Autodesk Fusion 360 part; units mm, degrees
(part 2 of 2)
  line L93 (-101.7927, 9.6669) -> (-102.2055, 10.4133)
  spline S43 degree 3 poles (-102.1987, 11.9336) (-102.3688, 11.6535) (-102.4812, 11.4913) (-102.5578, 11.3159) (-102.5705, 11.2723) (-102.5795, 11.182) (-102.5739, 11.1357) (-102.5157, 10.943) (-102.3981, 10.7613) (-102.2055, 10.4133) knots -0.305228 -0.305228 -0.305228 -0.305228 -0.202643 -0.202643 -0.163031 -0.163031 -0.119338 -0.119338 0 0 0 0
  line L94 (-102.1987, 11.9336) -> (-101.779, 12.625)
  line L95 (-101.779, 12.625) -> (-100.2331, 12.625)
  line L96 (-100.2331, 12.625) -> (-100.2331, 6.4783)
  spline S44 degree 3 poles (-78.8802, 8.0397) (-78.8802, 8.0397) (-78.8802, 8.0397) (-78.8801, 8.0397) (-78.8801, 8.0397) (-78.88, 8.0397) (-78.88, 8.0398) (-78.8798, 8.04) (-78.8797, 8.0402) (-78.8794, 8.041) (-78.8792, 8.0418) (-78.8786, 8.045) (-78.8782, 8.0484) (-78.8769, 8.0615) (-78.8761, 8.0763) (-78.8737, 8.1251) (-78.8722, 8.1818) (-78.8679, 8.3654) (-78.8655, 8.5656) (-78.8591, 9.2073) (-78.8573, 9.8073) (-78.8573, 10.3314) knots -0.220445 -0.220445 -0.220445 -0.220445 -0.220429 -0.220429 -0.220411 -0.220411 -0.220367 -0.220367 -0.220257 -0.220257 -0.219969 -0.219969 -0.219065 -0.219065 -0.216007 -0.216007 -0.203797 -0.203797 -0.157247 -0.157247 0 0 0 0
  spline S45 degree 3 poles (-79.66, 9.1105) (-79.3146, 8.6225) (-79.0132, 8.2063) (-78.9036, 8.0659) (-78.8903, 8.0491) (-78.8828, 8.0415) (-78.8818, 8.0406) (-78.8809, 8.0399) (-78.8807, 8.0398) (-78.8804, 8.0397) (-78.8803, 8.0397) (-78.8802, 8.0397) knots -0.01704 -0.01704 -0.01704 -0.01704 -0.001899 -0.001899 -0.000322 -0.000322 -0.000087 -0.000087 -0.000024 -0.000024 0 0 0 0
  line L97 (-79.66, 9.1105) -> (-80.4169, 10.1795)
  line L98 (-80.4169, 10.1795) -> (-80.4169, 12.6249)
  line L99 (-80.4169, 12.6249) -> (-78.8573, 12.6249)
  line L100 (-78.8573, 12.6249) -> (-78.8573, 10.3314)
  line L101 (-114.2466, 6.4942) -> (-115.0035, 6.4594)
  line L102 (-115.0035, 6.4594) -> (-115.0035, 7.2486)
  line L103 (-115.0035, 7.2486) -> (-115.0035, 8.0379)
  line L104 (-115.0035, 8.0379) -> (-114.5448, 8.0379)
  spline S46 degree 3 poles (-114.0861, 8.2672) (-114.0861, 8.2225) (-114.0874, 8.1854) (-114.0972, 8.1399) (-114.102, 8.1261) (-114.1159, 8.1022) (-114.1245, 8.0925) (-114.1483, 8.0745) (-114.1646, 8.0667) (-114.2516, 8.0407) (-114.362, 8.0379) (-114.5448, 8.0379) knots -0.128591 -0.128591 -0.128591 -0.128591 -0.100749 -0.100749 -0.086063 -0.086063 -0.071871 -0.071871 -0.054849 -0.054849 0 0 0 0
  spline S47 degree 3 poles (-113.2956, 8.4966) (-113.6377, 8.4966) (-113.8328, 8.4962) (-113.9744, 8.4707) (-113.9988, 8.4635) (-114.0318, 8.4477) (-114.0428, 8.44) (-114.0608, 8.4218) (-114.0676, 8.411) (-114.0856, 8.3666) (-114.0861, 8.3239) (-114.0861, 8.2672) knots -0.067797 -0.067797 -0.067797 -0.067797 -0.038062 -0.038062 -0.029608 -0.029608 -0.023495 -0.023495 -0.017016 -0.017016 0 0 0 0
  line L105 (-113.2956, 8.4966) -> (-112.5051, 8.4966)
  line L106 (-112.5051, 8.4966) -> (-112.543, 7.9012)
  spline S48 degree 3 poles (-114.2466, 6.4942) (-114.0442, 6.5035) (-113.8242, 6.522) (-113.4498, 6.5931) (-113.2959, 6.6391) (-113.052, 6.759) (-112.9528, 6.8282) (-112.7761, 7.0176) (-112.7103, 7.133) (-112.5965, 7.4348) (-112.5592, 7.6462) (-112.543, 7.9012) knots -0.314262 -0.314262 -0.314262 -0.314262 -0.243332 -0.243332 -0.182489 -0.182489 -0.132108 -0.132108 -0.076683 -0.076683 0 0 0 0
  line L107 (-103.9945, 6.4783) -> (-105.5541, 6.4783)
  line L108 (-105.5541, 6.4783) -> (-105.5511, 11.8451)
  line L109 (-105.5511, 11.8451) -> (-103.9945, 8.869)
  line L110 (-103.9945, 8.869) -> (-103.9945, 6.4783)
  line L111 (-79.6205, 6.4783) -> (-80.3728, 6.4783)
  line L112 (-80.3728, 6.4783) -> (-82.2755, 9.1431)
  spline S49 degree 3 poles (-84.1783, 12.22) (-84.1783, 12.1228) (-84.1718, 12.0391) (-84.0959, 11.8191) (-84.0269, 11.6832) (-83.6449, 11.0655) (-83.1484, 10.3655) (-82.2755, 9.1431) knots -0.89304 -0.89304 -0.89304 -0.89304 -0.671781 -0.671781 -0.450601 -0.450601 0 0 0 0
  line L113 (-84.1783, 12.22) -> (-84.1783, 12.6321)
  line L114 (-84.1783, 12.6321) -> (-83.3779, 12.6056)
  line L115 (-83.3779, 12.6056) -> (-82.5774, 12.5791)
  line L116 (-82.5774, 12.5791) -> (-80.7274, 9.9771)
  spline S50 degree 3 poles (-79.6205, 6.4783) (-79.3917, 6.4783) (-79.203, 6.4838) (-79.0027, 6.5232) (-78.949, 6.5392) (-78.8759, 6.5766) (-78.8498, 6.5945) (-78.8078, 6.6384) (-78.7925, 6.6625) (-78.7689, 6.7242) (-78.7644, 6.7611) (-78.7658, 6.8517) (-78.7776, 6.9137) (-78.9459, 7.4456) (-79.5495, 8.3203) (-80.7274, 9.9771) knots -1.178058 -1.178058 -1.178058 -1.178058 -0.964403 -0.964403 -0.875567 -0.875567 -0.82025 -0.82025 -0.769095 -0.769095 -0.704441 -0.704441 -0.609856 -0.609856 0 0 0 0
  line L117 (-62.7108, 11.0653) -> (-64.2704, 11.0653)
  line L118 (-64.2704, 11.0653) -> (-64.2704, 12.6249)
  line L119 (-64.2704, 12.6249) -> (-62.7108, 12.6249)
  line L120 (-62.7108, 12.6249) -> (-62.7108, 11.0653)
  line L121 (-85.4023, 6.4783) -> (-86.1675, 6.4783)
  line L122 (-86.1675, 6.4783) -> (-87.0995, 9.4403)
  spline S51 degree 3 poles (-87.2699, 12.625) (-87.4394, 12.625) (-87.5787, 12.6376) (-87.7375, 12.6363) (-87.7813, 12.6329) (-87.839, 12.6184) (-87.8597, 12.6108) (-87.894, 12.5891) (-87.9073, 12.5767) (-87.9308, 12.5439) (-87.9401, 12.5226) (-87.9545, 12.4632) (-87.9573, 12.4213) (-87.9358, 12.0193) (-87.6604, 11.2232) (-87.0995, 9.4403) knots -1.159539 -1.159539 -1.159539 -1.159539 -0.929801 -0.929801 -0.821044 -0.821044 -0.758836 -0.758836 -0.705055 -0.705055 -0.643157 -0.643157 -0.560713 -0.560713 0 0 0 0
  line L123 (-87.2699, 12.625) -> (-86.5083, 12.625)
  line L124 (-86.5083, 12.625) -> (-85.5727, 9.6479)
  spline S52 degree 3 poles (-84.637, 6.5745) (-84.637, 6.6129) (-84.8584, 7.3414) (-85.1118, 8.1738) (-85.3556, 8.9573) (-85.5727, 9.6479) knots -0.275208 -0.275208 -0.275208 -0.275208 -0.21716 -0.21716 0 0 0 0
  spline S53 degree 3 poles (-85.4023, 6.4783) (-85.1852, 6.4783) (-85.0047, 6.4859) (-84.8145, 6.507) (-84.7429, 6.5172) (-84.6801, 6.5376) (-84.666, 6.5432) (-84.6509, 6.5528) (-84.6464, 6.5562) (-84.6411, 6.5623) (-84.6395, 6.5648) (-84.6375, 6.5698) (-84.637, 6.5721) (-84.637, 6.5745) knots -0.053648 -0.053648 -0.053648 -0.053648 -0.020754 -0.020754 -0.006983 -0.006983 -0.003161 -0.003161 -0.001603 -0.001603 -0.000721 -0.000721 0 0 0 0
  line L125 (-45.0964, 6.4783) -> (-48.5826, 6.4783)
  line L126 (-48.5826, 6.4783) -> (-48.5826, 8.0379)
  line L127 (-48.5826, 8.0379) -> (-45.0964, 8.0379)
  line L128 (-45.0964, 8.0379) -> (-45.0964, 6.4783)
  line L129 (-115.3705, 6.4783) -> (-115.9897, 6.4865)
  spline S54 degree 3 poles (-116.9301, 6.5861) (-116.8418, 6.561) (-116.6918, 6.5372) (-116.3514, 6.5012) (-116.1605, 6.4888) (-115.9897, 6.4865) knots -0.102601 -0.102601 -0.102601 -0.102601 -0.051231 -0.051231 0 0 0 0
  spline S55 degree 3 poles (-117.8471, 9.57) (-117.8473, 8.4438) (-117.8321, 7.7752) (-117.7062, 7.2163) (-117.6651, 7.1041) (-117.5648, 6.9297) (-117.5053, 6.8604) (-117.3031, 6.7061) (-117.1405, 6.6459) (-116.9301, 6.5861) knots -0.278348 -0.278348 -0.278348 -0.278348 -0.149693 -0.149693 -0.105736 -0.105736 -0.065646 -0.065646 0 0 0 0
  spline S56 degree 3 poles (-116.1845, 12.6085) (-116.5349, 12.5917) (-116.8146, 12.5695) (-117.1517, 12.4821) (-117.2527, 12.4421) (-117.4251, 12.3326) (-117.4945, 12.2657) (-117.621, 12.084) (-117.6743, 11.9601) (-117.8311, 11.3627) (-117.847, 10.6695) (-117.8471, 9.57) knots -0.833641 -0.833641 -0.833641 -0.833641 -0.642856 -0.642856 -0.543072 -0.543072 -0.446446 -0.446446 -0.329868 -0.329868 0 0 0 0
  line L130 (-116.1845, 12.6085) -> (-115.3705, 12.6474)
  line L131 (-115.3705, 12.6474) -> (-115.3705, 11.0653)
  line L132 (-115.3705, 11.0653) -> (-116.2879, 11.0653)
  line L133 (-116.2879, 11.0653) -> (-116.2879, 8.0379)
  line L134 (-116.2879, 8.0379) -> (-115.3705, 8.0379)
  line L135 (-115.3705, 8.0379) -> (-115.3705, 6.4783)
  line L136 (-45.0964, 11.0653) -> (-48.5826, 11.0653)
  line L137 (-48.5826, 11.0653) -> (-48.5826, 12.6249)
  line L138 (-48.5826, 12.6249) -> (-45.0964, 12.6249)
  line L139 (-45.0964, 12.6249) -> (-45.0964, 11.0653)
  line L140 (-97.8478, 6.4783) -> (-99.4074, 6.4783)
  line L141 (-99.4074, 6.4783) -> (-99.4074, 12.625)
  line L142 (-99.4074, 12.625) -> (-97.8478, 12.625)
  line L143 (-97.8478, 12.625) -> (-97.8478, 10.3314)
  line L144 (-97.8478, 10.3314) -> (-95.5543, 10.3314)
  line L145 (-95.5543, 10.3314) -> (-95.5543, 8.7718)
  line L146 (-95.5543, 8.7718) -> (-97.8478, 8.7718)
  line L147 (-97.8478, 8.7718) -> (-97.8478, 6.4783)
  line L148 (-33.9039, 6.4783) -> (-35.4635, 6.4783)
  line L149 (-35.4635, 6.4783) -> (-35.4635, 12.625)
  line L150 (-35.4635, 12.625) -> (-33.9039, 12.625)
  line L151 (-33.9039, 12.625) -> (-33.9039, 6.4783)
  line L152 (-56.4723, 15.5607) -> (-68.9721, 15.5821)
  spline S57 degree 3 poles (-89.4076, 15.6509) (-86.7693, 15.6352) (-82.9576, 15.6207) (-76.5472, 15.5991) (-72.5191, 15.5882) (-68.9721, 15.5821) knots -1.903231 -1.903231 -1.903231 -1.903231 -1.064079 -1.064079 0 0 0 0
  line L153 (-89.4076, 15.6509) -> (-97.3432, 15.6983)
  line L154 (-97.3432, 15.6983) -> (-97.7592, 15.9429)
  spline S58 degree 3 poles (-99.1226, 17.4492) (-99.0892, 17.328) (-99.0113, 17.1818) (-98.789, 16.861) (-98.6488, 16.6966) (-98.2743, 16.3106) (-98.0079, 16.089) (-97.7592, 15.9429) knots -0.188555 -0.188555 -0.188555 -0.188555 -0.139214 -0.139214 -0.086539 -0.086539 0 0 0 0
  spline S59 degree 3 poles (-98.9864, 50.8517) (-98.9911, 50.8453) (-98.9953, 50.8331) (-99.0039, 50.8005) (-99.0081, 50.7769) (-99.0212, 50.6942) (-99.0295, 50.6103) (-99.0547, 50.3256) (-99.0704, 50.0212) (-99.1162, 49.0261) (-99.1433, 47.961) (-99.2165, 44.6686) (-99.2514, 41.4562) (-99.3158, 33.3141) (-99.3327, 25.6501) (-99.2383, 19.703) (-99.2057, 18.1555) (-99.141, 17.546) (-99.1325, 17.485) (-99.1226, 17.4492) knots -0.753543 -0.753543 -0.753543 -0.753543 -0.752585 -0.752585 -0.751244 -0.751244 -0.746826 -0.746826 -0.731243 -0.731243 -0.675641 -0.675641 -0.492875 -0.492875 -0.101584 -0.101584 -0.011142 -0.011142 0 0 0 0
  spline S60 degree 3 poles (-97.6115, 51.8685) (-97.7381, 51.8297) (-97.905, 51.7426) (-98.2587, 51.517) (-98.4433, 51.3796) (-98.7619, 51.1069) (-98.8991, 50.9696) (-98.9864, 50.8517) knots -0.133226 -0.133226 -0.133226 -0.133226 -0.088898 -0.088898 -0.04403 -0.04403 0 0 0 0
  line L155 (-97.6115, 51.8685) -> (-97.2974, 51.9649)
  line L156 (-97.2974, 51.9649) -> (-97.2974, 41.4318)
  line L157 (-97.2974, 41.4318) -> (-55.2594, 41.4318)
  line L158 (-55.2594, 41.4318) -> (-55.293, 43.7621)
  spline S61 degree 3 poles (-55.4873, 46.2701) (-55.4696, 46.2505) (-55.4537, 46.2289) (-55.4251, 46.175) (-55.4124, 46.1429) (-55.3771, 46.0158) (-55.3607, 45.8968) (-55.3207, 45.3803) (-55.3078, 44.7936) (-55.293, 43.7621) knots -0.596533 -0.596533 -0.596533 -0.596533 -0.525906 -0.525906 -0.45618 -0.45618 -0.309498 -0.309498 0 0 0 0
  spline S62 degree 3 poles (-69.4629, 46.5127) (-62.711, 46.481) (-58.3896, 46.4638) (-56.1245, 46.3995) (-55.8319, 46.3788) (-55.623, 46.3419) (-55.5805, 46.3307) (-55.519, 46.302) (-55.5025, 46.2868) (-55.4873, 46.2701) knots -0.093492 -0.093492 -0.093492 -0.093492 -0.034723 -0.034723 -0.014015 -0.014015 -0.006763 -0.006763 0 0 0 0
  line L159 (-69.4629, 46.5127) -> (-83.2775, 46.5775)
  line L160 (-83.2775, 46.5775) -> (-83.6132, 46.7899)
  spline S63 degree 3 poles (-85.3491, 48.778) (-85.019, 48.2927) (-84.6892, 47.8379) (-84.1216, 47.1878) (-83.8749, 46.9555) (-83.6132, 46.7899) knots -0.206339 -0.206339 -0.206339 -0.206339 -0.092903 -0.092903 0 0 0 0
  spline S64 degree 3 poles (-91.0655, 50.1326) (-88.6112, 50.1133) (-87.416, 50.1372) (-86.5601, 50.0031) (-86.4004, 49.9619) (-86.1321, 49.8336) (-86.0312, 49.7524) (-85.7647, 49.4518) (-85.6184, 49.1738) (-85.3491, 48.778) knots -0.584907 -0.584907 -0.584907 -0.584907 -0.300239 -0.300239 -0.220672 -0.220672 -0.143615 -0.143615 0 0 0 0
  line L161 (-91.0655, 50.1326) -> (-95.7377, 50.1693)
  line L162 (-95.7377, 50.1693) -> (-95.7377, 52.0799)
  line L163 (-95.7377, 52.0799) -> (-90.8066, 52.0539)
  spline S65 degree 3 poles (-83.8295, 49.9505) (-84.0958, 50.3279) (-84.3005, 50.6363) (-84.6712, 51.1429) (-84.8365, 51.3402) (-85.2066, 51.645) (-85.4099, 51.7541) (-86.4717, 52.0742) (-87.8185, 52.0382) (-90.8066, 52.0539) knots -1.794879 -1.794879 -1.794879 -1.794879 -1.492633 -1.492633 -1.191023 -1.191023 -0.896439 -0.896439 0 0 0 0
  spline S66 degree 3 poles (-82.8493, 48.6794) (-82.9472, 48.771) (-83.183, 49.0756) (-83.4316, 49.3979) (-83.6422, 49.685) (-83.8295, 49.9505) knots -0.125414 -0.125414 -0.125414 -0.125414 -0.097474 -0.097474 0 0 0 0
  line L164 (-82.8493, 48.6794) -> (-82.604, 48.45)
  line L165 (-82.604, 48.45) -> (-55.5091, 48.3583)
  line L166 (-55.5091, 48.3583) -> (-55.1061, 48.1434)
  spline S67 degree 3 poles (-53.6648, 46.8263) (-53.7712, 47.0322) (-54.0832, 47.362) (-54.6575, 47.8542) (-54.9064, 48.0368) (-55.1061, 48.1434) knots -0.164794 -0.164794 -0.164794 -0.164794 -0.0679 -0.0679 0 0 0 0
  spline S68 degree 3 poles (-53.3728, 31.2026) (-53.3681, 33.606) (-53.351, 40.3821) (-53.4152, 45.0538) (-53.4593, 45.9053) (-53.5693, 46.5942) (-53.6129, 46.726) (-53.6648, 46.8263) knots -0.214335 -0.214335 -0.214335 -0.214335 -0.10226 -0.10226 -0.033878 -0.033878 0 0 0 0
  line L167 (-53.3728, 31.2026) -> (-53.399, 17.7166)
  line L168 (-53.399, 17.7166) -> (-53.596, 17.3496)
  spline S69 degree 3 poles (-54.8891, 15.9513) (-54.6764, 16.0704) (-54.424, 16.2881) (-53.9545, 16.7958) (-53.7379, 17.0854) (-53.596, 17.3496) knots -0.179819 -0.179819 -0.179819 -0.179819 -0.089989 -0.089989 0 0 0 0
  line L169 (-54.8891, 15.9513) -> (-55.2563, 15.7456)
  line L170 (-55.2563, 15.7456) -> (-55.2956, 27.4879)
  spline S70 degree 3 poles (-55.4423, 39.3376) (-55.441, 39.3362) (-55.4397, 39.3342) (-55.4371, 39.3285) (-55.4359, 39.3248) (-55.4319, 39.3113) (-55.4294, 39.2983) (-55.4217, 39.2518) (-55.417, 39.2021) (-55.4026, 39.0273) (-55.3943, 38.8236) (-55.3691, 38.117) (-55.3562, 37.2035) (-55.3186, 34.1616) (-55.3002, 28.8469) (-55.2956, 27.4879) knots -0.518535 -0.518535 -0.518535 -0.518535 -0.518166 -0.518166 -0.517699 -0.517699 -0.516266 -0.516266 -0.511251 -0.511251 -0.49169 -0.49169 -0.407714 -0.407714 0 0 0 0
  spline S71 degree 3 poles (-97.1394, 39.3329) (-97.138, 39.3344) (-97.1361, 39.3356) (-97.132, 39.338) (-97.1293, 39.3392) (-97.1196, 39.3431) (-97.1109, 39.3456) (-97.0801, 39.3533) (-97.0496, 39.3582) (-96.9438, 39.3732) (-96.8314, 39.3825) (-96.4542, 39.4106) (-96.0393, 39.4275) (-94.6963, 39.4761) (-93.2418, 39.5024) (-88.7907, 39.5708) (-84.4694, 39.5949) (-72.6598, 39.6289) (-62.9423, 39.5936) (-57.2607, 39.4591) (-56.0416, 39.4239) (-55.5608, 39.3673) (-55.5023, 39.3593) (-55.461, 39.3472) (-55.4533, 39.3446) (-55.4458, 39.3404) (-55.4438, 39.3391) (-55.4423, 39.3376) knots -0.910234 -0.910234 -0.910234 -0.910234 -0.910118 -0.910118 -0.909959 -0.909959 -0.909514 -0.909514 -0.908106 -0.908106 -0.903203 -0.903203 -0.885257 -0.885257 -0.82008 -0.82008 -0.606432 -0.606432 -0.102188 -0.102188 -0.011575 -0.011575 -0.002565 -0.002565 -0.000642 -0.000642 0 0 0 0
  spline S72 degree 3 poles (-97.0853, 17.7179) (-97.0861, 17.7185) (-97.0868, 17.7193) (-97.0881, 17.7212) (-97.0888, 17.7224) (-97.0911, 17.727) (-97.0925, 17.7311) (-97.0967, 17.7454) (-97.0994, 17.7594) (-97.1083, 17.8129) (-97.1137, 17.8689) (-97.13, 18.0564) (-97.1401, 18.2645) (-97.1692, 18.9374) (-97.1859, 19.6709) (-97.2303, 21.9169) (-97.2496, 24.1113) (-97.2855, 30.2749) (-97.2759, 35.184) (-97.2108, 38.2563) (-97.1914, 38.9704) (-97.1577, 39.2596) (-97.1529, 39.2956) (-97.1454, 39.3213) (-97.1438, 39.3261) (-97.1412, 39.3307) (-97.1403, 39.332) (-97.1394, 39.3329) knots -0.457617 -0.457617 -0.457617 -0.457617 -0.457553 -0.457553 -0.457466 -0.457466 -0.457222 -0.457222 -0.456488 -0.456488 -0.454212 -0.454212 -0.445793 -0.445793 -0.414977 -0.414977 -0.313166 -0.313166 -0.061484 -0.061484 -0.007183 -0.007183 -0.001603 -0.001603 -0.000403 -0.000403 0 0 0 0
  spline S73 degree 3 poles (-75.6693, 17.5007) (-76.728, 17.4989) (-87.3101, 17.4779) (-94.5713, 17.5117) (-96.0081, 17.5427) (-96.8124, 17.6286) (-96.9225, 17.65) (-97.0357, 17.6879) (-97.0642, 17.7025) (-97.0853, 17.7179) knots -0.139613 -0.139613 -0.139613 -0.139613 -0.07072 -0.07072 -0.021621 -0.021621 -0.007859 -0.007859 0 0 0 0
  line L171 (-75.6693, 17.5007) -> (-56.4723, 17.5331)
  line L172 (-56.4723, 17.5331) -> (-56.4723, 16.5469)
  line L173 (-56.4723, 16.5469) -> (-56.4723, 15.5607)
  line L174 (-55.0962, 6.4783) -> (-56.6558, 6.4783)
  line L175 (-56.6558, 6.4783) -> (-56.6558, 12.625)
  line L176 (-56.6558, 12.625) -> (-55.0962, 12.625)
  line L177 (-55.0962, 12.625) -> (-55.0962, 6.4783)
  line L178 (-94.0864, 11.0653) -> (-97.5726, 11.0653)
  line L179 (-97.5726, 11.0653) -> (-97.5726, 12.6249)
  line L180 (-97.5726, 12.6249) -> (-94.0864, 12.6249)
  line L181 (-94.0864, 12.6249) -> (-94.0864, 11.0653)
  line L182 (-74.8895, 6.4941) -> (-76.105, 6.4641)
  line L183 (-76.105, 6.4641) -> (-76.105, 8.0379)
  line L184 (-76.105, 8.0379) -> (-74.2702, 8.0379)
  line L185 (-74.2702, 8.0379) -> (-74.2702, 11.0653)
  line L186 (-74.2702, 11.0653) -> (-76.105, 11.0653)
  line L187 (-76.105, 11.0653) -> (-76.105, 12.625)
  line L188 (-76.105, 12.625) -> (-74.9553, 12.625)
  spline S74 degree 3 poles (-72.9858, 12.125) (-73.0813, 12.2284) (-73.1739, 12.3119) (-73.3849, 12.446) (-73.5011, 12.495) (-73.9311, 12.6041) (-74.3272, 12.625) (-74.9553, 12.625) knots -0.375116 -0.375116 -0.375116 -0.375116 -0.281955 -0.281955 -0.188436 -0.188436 0 0 0 0
  line L189 (-72.9858, 12.125) -> (-72.7565, 11.8766)
  line L190 (-72.7565, 11.8766) -> (-72.7291, 9.6563)
  spline S75 degree 3 poles (-74.8895, 6.4941) (-74.4917, 6.5039) (-74.1599, 6.5143) (-73.6854, 6.5676) (-73.5163, 6.6021) (-73.2815, 6.6935) (-73.1934, 6.7421) (-73.0348, 6.88) (-72.9733, 6.9649) (-72.8626, 7.1876) (-72.8183, 7.3432) (-72.7133, 7.9996) (-72.717, 8.6759) (-72.7291, 9.6563) knots -0.902906 -0.902906 -0.902906 -0.902906 -0.730286 -0.730286 -0.599267 -0.599267 -0.510748 -0.510748 -0.416898 -0.416898 -0.294122 -0.294122 0 0 0 0
  line L191 (-88.3645, 6.5241) -> (-89.1725, 6.4975)
  spline S76 degree 3 poles (-89.9398, 6.5892) (-89.942, 6.5829) (-89.9435, 6.5761) (-89.9434, 6.5644) (-89.9425, 6.5596) (-89.9386, 6.5498) (-89.9354, 6.5452) (-89.9255, 6.5351) (-89.9178, 6.5301) (-89.8862, 6.5148) (-89.8516, 6.5068) (-89.6863, 6.487) (-89.4867, 6.4871) (-89.1725, 6.4975) knots -0.177308 -0.177308 -0.177308 -0.177308 -0.165649 -0.165649 -0.157054 -0.157054 -0.147301 -0.147301 -0.132691 -0.132691 -0.094301 -0.094301 0 0 0 0
  spline S77 degree 3 poles (-89.1259, 9.206) (-89.3376, 8.5218) (-89.6008, 7.6731) (-89.818, 6.9764) (-89.9278, 6.6244) (-89.9398, 6.5892) knots -0.080263 -0.080263 -0.080263 -0.080263 -0.011151 -0.011151 0 0 0 0
  spline S78 degree 3 poles (-88.3067, 11.7047) (-88.3068, 11.7047) (-88.3069, 11.7046) (-88.3071, 11.7046) (-88.3072, 11.7045) (-88.3076, 11.7043) (-88.3079, 11.7041) (-88.3088, 11.7032) (-88.3094, 11.7023) (-88.3118, 11.6988) (-88.3137, 11.6951) (-88.3207, 11.6807) (-88.3273, 11.6646) (-88.3486, 11.6111) (-88.3706, 11.5496) (-88.4414, 11.349) (-88.5135, 11.1314) (-88.7428, 10.4319) (-88.9486, 9.7787) (-89.1259, 9.206) knots -0.253396 -0.253396 -0.253396 -0.253396 -0.25335 -0.25335 -0.253297 -0.253297 -0.253158 -0.253158 -0.252762 -0.252762 -0.251615 -0.251615 -0.2479 -0.2479 -0.233576 -0.233576 -0.179867 -0.179867 0 0 0 0
  spline S79 degree 3 poles (-87.7004, 9.8026) (-87.9497, 10.6489) (-88.1764, 11.3726) (-88.2771, 11.644) (-88.2904, 11.6786) (-88.3007, 11.6978) (-88.3024, 11.7008) (-88.3045, 11.7033) (-88.305, 11.7038) (-88.3057, 11.7044) (-88.306, 11.7045) (-88.3064, 11.7046) (-88.3065, 11.7047) (-88.3067, 11.7047) knots -0.041282 -0.041282 -0.041282 -0.041282 -0.004966 -0.004966 -0.000968 -0.000968 -0.000317 -0.000317 -0.000127 -0.000127 -0.000047 -0.000047 0 0 0 0
  line L192 (-87.7004, 9.8026) -> (-87.14, 7.9003)
  line L193 (-87.14, 7.9003) -> (-87.9805, 7.8085)
  line L194 (-87.9805, 7.8085) -> (-88.3645, 6.5241)
  line L195 (-82.6187, 6.4783) -> (-84.1783, 6.4783)
  line L196 (-84.1783, 6.4783) -> (-84.1783, 8.7718)
  spline S80 degree 3 poles (-84.1377, 11.0653) (-84.1378, 11.0653) (-84.1379, 11.0653) (-84.138, 11.0653) (-84.1381, 11.0652) (-84.1384, 11.065) (-84.1386, 11.0648) (-84.1391, 11.064) (-84.1395, 11.0632) (-84.1406, 11.06) (-84.1413, 11.0565) (-84.1435, 11.0439) (-84.1448, 11.0303) (-84.1492, 10.9794) (-84.1519, 10.9227) (-84.1595, 10.7387) (-84.1638, 10.5385) (-84.1752, 9.8963) (-84.1783, 9.2962) (-84.1783, 8.7718) knots -0.221851 -0.221851 -0.221851 -0.221851 -0.221787 -0.221787 -0.221717 -0.221717 -0.221546 -0.221546 -0.221114 -0.221114 -0.219931 -0.219931 -0.216241 -0.216241 -0.203961 -0.203961 -0.15732 -0.15732 0 0 0 0
  spline S81 degree 3 poles (-83.3579, 10.0354) (-83.6735, 10.4751) (-83.9559, 10.8533) (-84.0957, 11.0232) (-84.1168, 11.048) (-84.1309, 11.0611) (-84.1333, 11.0632) (-84.1358, 11.0647) (-84.1364, 11.0651) (-84.1372, 11.0653) (-84.1374, 11.0653) (-84.1377, 11.0653) knots -0.026824 -0.026824 -0.026824 -0.026824 -0.004356 -0.004356 -0.000837 -0.000837 -0.000243 -0.000243 -0.000072 -0.000072 0 0 0 0
  line L197 (-83.3579, 10.0354) -> (-82.6187, 9.0054)
  line L198 (-82.6187, 9.0054) -> (-82.6187, 6.4783)
  line L199 (-60, 85) -> (-25, 0)
  line L200 (-125, 0) -> (-95, 85)
  constraint coincident L3 L199.start
  constraint coincident L1.end L2.start
  constraint coincident L0.end L1.start
  constraint coincident L3 L200.end
extrude "Extrude8" cut sketch "Sketch3" against normal blind 5 contours L0 L3 L200 | L2 L3 L199
